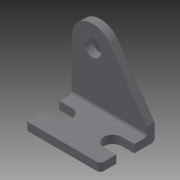
# Autodesk Inventor part: D-168
Saved by Autodesk Inventor 2014 (Build 180170000, 170)
## iProperties
Created: 2014-01-18
Part Number: D-168
Material: Generic
Catalog Web Link: www.cadenas.de
Description: Pivot Bracket for Original Line Cylinders - Left-
Vendor: BIMBA
Document SubType Name: Standard Catalog Part
Designer: Andrew Toennies
Manufacturer: BIMBA
Density: 1 g/cm^3
Appearance: RGB(192.00000375509219,192.00000375509219,192.00000375509219)
Category: PARTsolutions
Company: BIMBA
Title: D-168
Author: Cadenas PARTsolutions
PSOL_IDENT_0: {$CADENAS_DATA\23d-libs\bimba\bimba\bimba_imperial\bimba_full_line\original_line_cylinders\accessori
PSOL_IDENT_1: es\pivot_bracket_left.prj},194 {VTYP=3D},{NB=D-168},{LINA=D-168},{NN=Pivot Bracket for Original Line
PSOL_IDENT_2: Cylinders - Left},{DATE=09.12.2011 06:37:01},{GEOMDATE=09.12.2011 06:36:00},{VERSION=},{LINEID=30},
PSOL_IDENT_3: {LINESUBID=-1},{WBVAR=}  {NB=D-168},{LINA=D-168},{KT=DUMMY},{PN=D-168},{MAT=Zinc-Plated Carbon Steel
PSOL_IDENT_4: },{CD=0},{L=1.12500000},{L1=0.75000000},{L2=0.37500000},{L3=0.56250000},{L5=0.31300000},{L6=0.119600
PSOL_IDENT_5: 00},{H=1.19000000},{H1=0.25000000},{H2=0.87500000},{H22=0.875},{W=0.81700000},{W1=0.27000000},{W2=0.
PSOL_IDENT_6: 44050000},{R1=0.13500000},{R2=0.31300000},{R3=0.05000000},{D1=0.25275000},{C=1}
CNS_NN: Pivot Bracket for Original Line Cylinders - Left
CNS_NB: D-168
CNS_NBSYN: $PN.
CNS_LINA: D-168
CNS_PN: D-168
CNS_MAT: Zinc-Plated Carbon Steel
CNS_CD: 0
CNS_L: 1.12500000
CNS_L1: 0.75000000
CNS_L2: 0.37500000
CNS_L3: 0.56250000
CNS_L5: 0.31300000
CNS_L6: 0.11960000
CNS_H: 1.19000000
CNS_H1: 0.25000000
CNS_H2: 0.87500000
CNS_H22: 0.875
CNS_W: 0.81700000
CNS_W1: 0.27000000
CNS_W2: 0.44050000
CNS_R1: 0.13500000
CNS_R2: 0.31300000
CNS_R3: 0.05000000
CNS_D1: 0.25275000
CNS_C: 1
SUPPLIER: BIMBA
ARTICLENO: D-168
BOMINFO: D-168
CREATOR: CADENAS GmbH
Autodesk Inventor part; units mm, degrees
ref_plane "YZ Plane" through (0, 0, 0) normal (1, 0, 0) x (0, 1, 0)
ref_plane "XZ Plane" through (0, 0, 0) normal (0, 1, 0) x (-1, 0, 0)
ref_plane "XY Plane" through (0, 0, 0) normal (0, 0, 1) x (1, 0, 0)
sketch "Sketch_1" plane through (0, 0, 0) normal (1, 0, 0) x (0, 1, 0)
  line L0 (0, 20.7518) -> (0, 1.27)
  arc A0 (0, 1.27) -> (1.27, 0) centre (1.27, 1.27) ccw
  line L1 (1.27, 0) -> (30.226, 0)
  line L2 (30.226, 0) -> (30.226, 3.0378)
  line L3 (30.226, 3.0378) -> (4.3078, 3.0378)
  arc A1 (3.0378, 4.3078) -> (4.3078, 3.0378) centre (4.3078, 4.3078) ccw
  line L4 (3.0378, 4.3078) -> (3.0378, 20.7518)
  line L5 (3.0378, 20.7518) -> (0, 20.7518)
  constraints: 12 end point, 4 point on circle, 2 centre point
extrude "Extrusion1" add sketch "Sketch_1" along normal blind 28.575
sketch "Sketch_2" plane through (0, 0, 0) normal (0, 0, 1) x (1, 0, 0)
  line L0 (-28.575, -30.226) -> (42.8625, -30.226)
  line L1 (42.8625, -30.226) -> (42.8625, 45.339)
  line L2 (42.8625, 45.339) -> (-28.575, 45.339)
  line L3 (-28.575, 45.339) -> (-28.575, -30.226)
  line L4 (0, 0) -> (28.575, 0)
  line L5 (28.575, 0) -> (28.575, 6.35)
  line L6 (28.575, 6.35) -> (14.4921, 26.7427)
  arc A0 (14.4921, 26.7427) -> (0, 22.225) centre (7.9502, 22.225) ccw
  line L7 (0, 22.225) -> (0, 0)
  constraints: 16 end point, 2 point on circle, 1 centre point
extrude "Extrusion2" cut sketch "Sketch_2" along normal blind 20.7518
sketch "Sketch3" plane through (28.575, 1.27, 0) normal (0, 0, -1) x (-1, 0, 0)
  point P0 (20.6248, 20.955)
hole "Hole1" at (7.9502, 22.225, 0) direction (0, 0, 1) diameter 6.4198 depth 3.0378
sketch "Sketch4" plane through (0, 0, 1.27) normal (0, -1, 0) x (1, 0, 0)
  point P0 (4.7625, 9.9187)
hole "Hole2" at (4.7625, 0, 11.1887) direction (0, 1, 0) diameter 6.858 depth 3.0378
sketch "Sketch5" plane through (0, 0, 1.27) normal (0, -1, 0) x (1, 0, 0)
  point P0 (23.8125, 9.9187)
hole "Hole3" at (23.8125, 0, 11.1887) direction (0, 1, 0) diameter 6.858 depth 3.0378
sketch "Sketch_6" plane through (0, 0, 0) normal (0, 1, 0) x (-1, 0, 0)
  line L0 (0, 7.7597) -> (0, 14.6177)
  line L1 (0, 14.6177) -> (-4.7625, 14.6177)
  line L2 (-4.7625, 14.6177) -> (-4.7625, 7.7597)
  line L3 (-4.7625, 7.7597) -> (0, 7.7597)
  constraints: 8 end point
sketch "Sketch_7" plane through (0, 0, 0) normal (0, 1, 0) x (-1, 0, 0)
  line L0 (-23.8125, 7.7597) -> (-23.8125, 14.6177)
  line L1 (-23.8125, 14.6177) -> (-28.575, 14.6177)
  line L2 (-28.575, 14.6177) -> (-28.575, 7.7597)
  line L3 (-28.575, 7.7597) -> (-23.8125, 7.7597)
  constraints: 8 end point
extrude "Extrusion3" cut sketch "Sketch_6" along normal blind 3.0378
extrude "Extrusion4" cut sketch "Sketch_7" along normal blind 3.0378
sketch "Sketch_8" plane through (0, 0, 0) normal (0, 1, 0) x (-1, 0, 0)
  line L0 (0, 31.1277) -> (-28.575, 31.1277)
  line L1 (-28.575, 31.1277) -> (-28.575, 19.4818)
  arc A0 (-27.305, 20.7518) -> (-28.575, 19.4818) centre (-27.305, 19.4818) ccw
  line L2 (-27.305, 20.7518) -> (-1.27, 20.7518)
  arc A1 (0, 19.4818) -> (-1.27, 20.7518) centre (-1.27, 19.4818) ccw
  line L3 (0, 19.4818) -> (0, 31.1277)
  constraints: 8 end point, 4 point on circle, 2 centre point
extrude "Extrusion5" cut sketch "Sketch_8" along normal blind 3.0378
ref_plane "a1_XY" through (0, 22.225, 0) normal (0, 0, 1) x (1, 0, 0)
ref_plane "a1_YZ" through (0, 22.225, 0) normal (1, 0, 0) x (0, 1, 0)
ref_plane "a1_ZX" through (0, 22.225, 0) normal (0, 1, 0) x (0, 0, 1)
ref_plane "a2_XY" through (7.9502, 22.225, 0) normal (0, 0, 1) x (1, 0, 0)
ref_plane "a2_YZ" through (7.9502, 22.225, 0) normal (1, 0, 0) x (0, 1, 0)
ref_plane "a2_ZX" through (7.9502, 22.225, 0) normal (0, 1, 0) x (0, 0, 1)
ref_plane "b1_XY" through (4.7403, 22.225, 0) normal (0, 0, 1) x (1, 0, 0)
ref_plane "b1_YZ" through (4.7403, 22.225, 0) normal (1, 0, 0) x (0, 1, 0)
ref_plane "b1_ZX" through (4.7403, 22.225, 0) normal (0, 1, 0) x (0, 0, 1)
ref_plane "b2_XY" through (11.1601, 22.225, 0) normal (0, 0, 1) x (1, 0, 0)
ref_plane "b2_YZ" through (11.1601, 22.225, 0) normal (1, 0, 0) x (0, 1, 0)
ref_plane "b2_ZX" through (11.1601, 22.225, 0) normal (0, 1, 0) x (0, 0, 1)
ref_plane "d1_XY" through (0, 30.226, 0) normal (1, 0, 0) x (0, 0, -1)
ref_plane "d1_YZ" through (0, 30.226, 0) normal (0, 0, -1) x (0, 1, 0)
ref_plane "d1_ZX" through (0, 30.226, 0) normal (0, 1, 0) x (1, 0, 0)
ref_plane "d2_XY" through (0, 30.226, 3.0378) normal (1, 0, 0) x (0, 0, -1)
ref_plane "d2_YZ" through (0, 30.226, 3.0378) normal (0, 0, -1) x (0, 1, 0)
ref_plane "d2_ZX" through (0, 30.226, 3.0378) normal (0, 1, 0) x (1, 0, 0)
ref_plane "e1_XY" through (0, 0, 0) normal (0, 0, 1) x (1, 0, 0)
ref_plane "e1_YZ" through (0, 0, 0) normal (1, 0, 0) x (0, 1, 0)
ref_plane "e1_ZX" through (0, 0, 0) normal (0, 1, 0) x (0, 0, 1)
ref_plane "e2_XY" through (7.9502, 30.1752, 0) normal (0, 0, 1) x (1, 0, 0)
ref_plane "e2_YZ" through (7.9502, 30.1752, 0) normal (1, 0, 0) x (0, 1, 0)
ref_plane "e2_ZX" through (7.9502, 30.1752, 0) normal (0, 1, 0) x (0, 0, 1)
ref_plane "f1_XY" through (0, 0, 0) normal (0, 0, 1) x (1, 0, 0)
ref_plane "f1_YZ" through (0, 0, 0) normal (1, 0, 0) x (0, 1, 0)
ref_plane "f1_ZX" through (0, 0, 0) normal (0, 1, 0) x (0, 0, 1)
ref_plane "f2_XY" through (0, 22.225, 0) normal (0, 0, 1) x (1, 0, 0)
ref_plane "f2_YZ" through (0, 22.225, 0) normal (1, 0, 0) x (0, 1, 0)
ref_plane "f2_ZX" through (0, 22.225, 0) normal (0, 1, 0) x (0, 0, 1)
ref_plane "g1_XY" through (0, 0, 7.7597) normal (0, 1, 0) x (1, 0, 0)
ref_plane "g1_YZ" through (0, 0, 7.7597) normal (1, 0, 0) x (0, 0, -1)
ref_plane "g1_ZX" through (0, 0, 7.7597) normal (0, 0, -1) x (0, 1, 0)
ref_plane "g2_XY" through (0, 0, 14.6177) normal (0, 1, 0) x (1, 0, 0)
ref_plane "g2_YZ" through (0, 0, 14.6177) normal (1, 0, 0) x (0, 0, -1)
ref_plane "g2_ZX" through (0, 0, 14.6177) normal (0, 0, -1) x (0, 1, 0)
ref_plane "h1_XY" through (4.7625, 0, 20.7518) normal (0, 0, 1) x (1, 0, 0)
ref_plane "h1_YZ" through (4.7625, 0, 20.7518) normal (1, 0, 0) x (0, 1, 0)
ref_plane "h1_ZX" through (4.7625, 0, 20.7518) normal (0, 1, 0) x (0, 0, 1)
ref_plane "h2_XY" through (23.8125, 0, 20.7518) normal (0, 0, 1) x (1, 0, 0)
ref_plane "h2_YZ" through (23.8125, 0, 20.7518) normal (1, 0, 0) x (0, 1, 0)
ref_plane "h2_ZX" through (23.8125, 0, 20.7518) normal (0, 1, 0) x (0, 0, 1)
ref_plane "i_XY" through (28.575, 0, 20.7518) normal (0, 0, 1) x (1, 0, 0)
ref_plane "i_YZ" through (28.575, 0, 20.7518) normal (1, 0, 0) x (0, 1, 0)
ref_plane "i_ZX" through (28.575, 0, 20.7518) normal (0, 1, 0) x (0, 0, 1)
ref_plane "j1_XY" through (0, 0, 0) normal (0, 0, 1) x (1, 0, 0)
ref_plane "j1_YZ" through (0, 0, 0) normal (1, 0, 0) x (0, 1, 0)
ref_plane "j1_ZX" through (0, 0, 0) normal (0, 1, 0) x (0, 0, 1)
ref_plane "j2_XY" through (28.575, 0, 0) normal (0, 0, 1) x (1, 0, 0)
ref_plane "j2_YZ" through (28.575, 0, 0) normal (1, 0, 0) x (0, 1, 0)
ref_plane "j2_ZX" through (28.575, 0, 0) normal (0, 1, 0) x (0, 0, 1)
ref_plane "k11_XY" through (0, 0, 20.7518) normal (1, 0, 0) x (0, 0, -1)
ref_plane "k11_YZ" through (0, 0, 20.7518) normal (0, 0, -1) x (0, 1, 0)
ref_plane "k11_ZX" through (0, 0, 20.7518) normal (0, 1, 0) x (1, 0, 0)
ref_plane "k12_XY" through (0, 0, 0) normal (1, 0, 0) x (0, 0, -1)
ref_plane "k12_YZ" through (0, 0, 0) normal (0, 0, -1) x (0, 1, 0)
ref_plane "k12_ZX" through (0, 0, 0) normal (0, 1, 0) x (1, 0, 0)
ref_plane "to_dummy_L_XY" through (0, 0, 0) normal (0, 0, 1) x (1, 0, 0)
ref_plane "to_dummy_L_YZ" through (0, 0, 0) normal (1, 0, 0) x (0, 1, 0)
ref_plane "to_dummy_L_ZX" through (0, 0, 0) normal (0, 1, 0) x (0, 0, 1)
ref_plane "to_pin_L_XY" through (7.9502, 22.225, 0) normal (0, 0, 1) x (1, 0, 0)
ref_plane "to_pin_L_YZ" through (7.9502, 22.225, 0) normal (1, 0, 0) x (0, 1, 0)
ref_plane "to_pin_L_ZX" through (7.9502, 22.225, 0) normal (0, 1, 0) x (0, 0, 1)
body "Solid1"
